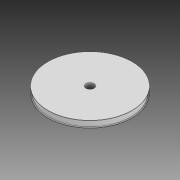
# Autodesk Inventor part: fakepully
Saved by Autodesk Inventor 2020 (Build 240168000, 168)
## iProperties
Created: 2021-04-24
Part Number: fakepully
Material: Generic
Document SubType Name: Modeling
Designer: DDeGo
Density: 1 g/cm^3
Appearance: Default
Author: DDeGo
Autodesk Inventor part; units mm, degrees
ref_plane "YZ Plane" through (0, 0, 0) normal (1, 0, 0) x (0, 1, 0)
ref_plane "XZ Plane" through (0, 0, 0) normal (0, 1, 0) x (-1, 0, 0)
ref_plane "XY Plane" through (0, 0, 0) normal (0, 0, 1) x (1, 0, 0)
sketch "Sketch1" plane through (0, 0, 0) normal (0, 0, 1) x (1, 0, 0)
  line L0 (0, 0) -> (-103, 0)
  line L1 (-103, 0) -> (-103, 1)
  line L2 (-103, 1) -> (-100, 1)
  line L3 (-100, 1) -> (-100, 16)
  line L4 (-100, 16) -> (-103, 16)
  line L5 (-103, 16) -> (-103, 17)
  line L6 (-103, 17) -> (-10, 17)
  line L7 (-10, 17) -> (-10, 0)
  line L8 (0, 0) -> (0, 15.4715) construction
  dimension "d0" = 100
  dimension "d1" = 15
  dimension "d2" = 1
  dimension "d3" = 1
  dimension "d4" = 10
  dimension "d5" = 3
  constraints: 18 end point, 5 perpendicular, 3 point on line, 2 vertical, 1 horizontal
  measures "d0" distance between parallel lines of L8 L3
  measures "d1" distance of L2.end L3.end
  measures "d2" distance of L4.end L5.end
  measures "d3" distance of L0.end L1.end
  measures "d4" distance between parallel lines of L8 L7
  measures "d5" distance between parallel lines of L5 L3
revolve "Revolution1" add sketch "Sketch1" angle 360 about axis through (0, 0, 0) along (0, 1, 0)
body "Solid1"
